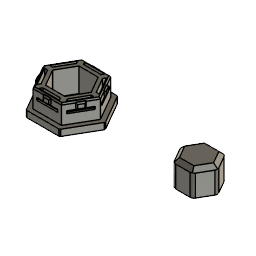
Inserts (Autodesk Fusion 360 design; units mm, degrees)
part number: 2025-05-12-14-06-05-452
part number: 2025-05-25-10-33-36-261
part number: 2025-05-25-10-36-06-309
Autodesk Fusion 360 part; units mm, degrees
sketch "Sketch1" plane through (0, 0, 0) normal (0, 0, 1) x (1, 0, 0)
  line L0 (-6.5818, 11.4) -> (-13.1636, 0)
  line L1 (-13.1636, 0) -> (-6.5818, -11.4)
  line L2 (-6.5818, -11.4) -> (6.5818, -11.4)
  line L3 (6.5818, -11.4) -> (13.1636, 0)
  line L4 (13.1636, 0) -> (6.5818, 11.4)
  line L5 (6.5818, 11.4) -> (-6.5818, 11.4)
  dimension "d1" = 11.4
  measures "d1" distance of origin L5
extrude "Extrude1" add sketch "Sketch1" along normal blind 2.5 makes body 1
sketch "Sketch2" plane through (0, 0, 2.5) normal (0, 0, 1) x (-1, 0, 0)
  line L0 (-6.5818, -11.4) -> (6.5818, -11.4)
  line L1 (6.5818, -11.4) -> (13.1636, 0)
  line L2 (13.1636, 0) -> (6.5818, 11.4)
  line L3 (6.5818, 11.4) -> (-6.5818, 11.4)
  line L4 (-6.5818, 11.4) -> (-13.1636, 0)
  line L5 (-13.1636, 0) -> (-6.5818, -11.4)
  line L6 (5.6003, -9.7) -> (11.2006, 0)
  line L7 (11.2006, 0) -> (5.6003, 9.7)
  line L8 (5.6003, 9.7) -> (-5.6003, 9.7)
  line L9 (-5.6003, 9.7) -> (-11.2006, 0)
  line L10 (-11.2006, 0) -> (-5.6003, -9.7)
  line L11 (-5.6003, -9.7) -> (5.6003, -9.7)
  dimension "d4" = 9.7
  measures "d4" distance of origin L11
extrude "Extrude2" add sketch "Sketch2" along normal blind 7.4 contours L6 L7 L8 L9 L10 L11 bodies 1
sketch "Sketch3" plane through (0, 0, 9.9) normal (0, 0, 1) x (-1, 0, 0)
  line L0 (-5.6003, -9.7) -> (5.6003, -9.7)
  line L1 (5.6003, -9.7) -> (11.2006, 0)
  line L2 (11.2006, 0) -> (5.6003, 9.7)
  line L3 (5.6003, 9.7) -> (-5.6003, 9.7)
  line L4 (-5.6003, 9.7) -> (-11.2006, 0)
  line L5 (-11.2006, 0) -> (-5.6003, -9.7)
  line L6 (3.7816, -6.55) -> (7.5633, 0)
  line L7 (7.5633, 0) -> (3.7816, 6.55)
  line L8 (3.7816, 6.55) -> (-3.7816, 6.55)
  line L9 (-3.7816, 6.55) -> (-7.5633, 0)
  line L10 (-7.5633, 0) -> (-3.7816, -6.55)
  line L11 (-3.7816, -6.55) -> (3.7816, -6.55)
  dimension "d7" = 6.55
  measures "d7" distance of origin L11
extrude "Extrude3" cut sketch "Sketch3" against normal up to surface (9.9 mm away) contours L6 L7 L8 L9 L10 L11 bodies 1
sketch "Sketch4" plane through (0, 0, 9.9) normal (0, 0, 1) x (-1, 0, 0)
  line L0 (-7.5633, 0) -> (-3.7816, 6.55)
  line L1 (-3.7816, 6.55) -> (3.7816, 6.55)
  line L2 (3.7816, 6.55) -> (7.5633, 0)
  line L3 (7.5633, 0) -> (3.7816, -6.55)
  line L4 (3.7816, -6.55) -> (-3.7816, -6.55)
  line L5 (-3.7816, -6.55) -> (-7.5633, 0)
  line L6 (-5.6003, -9.7) -> (5.6003, -9.7)
  line L7 (5.6003, -9.7) -> (11.2006, 0)
  line L8 (11.2006, 0) -> (5.6003, 9.7)
  line L9 (5.6003, 9.7) -> (-5.6003, 9.7)
  line L10 (-5.6003, 9.7) -> (-11.2006, 0)
  line L11 (-11.2006, 0) -> (-5.6003, -9.7)
  line L12 (11.2006, 0) -> (-11.2006, 0) construction
  line L13 (-5.6003, 9.7) -> (5.6003, -9.7) construction
  line L14 (-5.6292, -9.75) -> (5.6292, 9.75) construction
  line L15 (-3.4253, 7.9485) -> (3.431, 7.95)
  line L16 (3.431, 7.95) -> (4.0005, 8.9501)
  line L17 (4.0005, 8.9501) -> (-3.9995, 8.9484)
  line L18 (-3.9995, 8.9484) -> (-3.4253, 7.9485)
  line L19 (3.4049, -7.95) -> (-3.4457, -7.9788)
  line L20 (-3.4457, -7.9788) -> (-4.0185, -8.9812)
  line L21 (-4.0185, -8.9812) -> (3.9815, -8.9476)
  line L22 (3.9815, -8.9476) -> (3.4049, -7.95)
  line L23 (5.1681, 6.9487) -> (8.5549, 0.9746)
  line L24 (8.5549, 0.9746) -> (9.6988, 0.9846)
  line L25 (9.6988, 0.9846) -> (5.7533, 7.944)
  line L26 (5.7533, 7.944) -> (5.1681, 6.9487)
  line L27 (-9.6706, 0.9703) -> (-8.5268, 0.965)
  line L28 (-8.5268, 0.965) -> (-5.1652, 6.9536)
  line L29 (-5.7547, 7.9464) -> (-9.6706, 0.9703)
  line L30 (-5.1652, 6.9536) -> (-5.7547, 7.9464)
  line L31 (-5.1141, -6.9101) -> (-8.6037, -0.9979)
  line L32 (-8.6037, -0.9979) -> (-9.7575, -1.0105)
  line L33 (-9.7575, -1.0105) -> (-5.6911, -7.8999)
  line L34 (-5.6911, -7.8999) -> (-5.1141, -6.9101)
  line L35 (8.5998, -1.0047) -> (5.1477, -6.9347)
  line L36 (9.7535, -1.0105) -> (8.5998, -1.0047)
  line L37 (5.7287, -7.9243) -> (9.7535, -1.0105)
  line L38 (5.1477, -6.9347) -> (5.7287, -7.9243)
  point P0 (-0.0307, 8.5259)
  dimension "d10" = 8
  dimension "d11" = 1
  dimension "d12" = 6.8563
  dimension "d13" = 0.339
  dimension "d14" = 1.4
  dimension "d15" = 8
  dimension "d16" = 1
  dimension "d18" = 1.4
  dimension "d19" = 8
  dimension "d20" = 1
  dimension "d22" = 1.4
  dimension "d23" = 1.0105
  dimension "d24" = 1.0105
  dimension "d25" = 1.0105
  dimension "d26" = 1.0105
  dimension "d27" = 8
  dimension "d28" = 1
  dimension "d30" = 1.4
  dimension "d31" = 1.0105
  dimension "d32" = 8
  dimension "d33" = 1
  dimension "d35" = 1.4
  dimension "d36" = 1.0105
  dimension "d37" = 8
  dimension "d38" = 1
  dimension "d40" = 1.4
  dimension "d41" = 1.0105
  constraint coincident L7.end L8.start
  constraint coincident L10.end L11.start
  constraint coincident L9.end L10.start
  constraint coincident L6.end L7.start
  constraint coincident L6.start L11.end
  constraint coincident L8.end L9.start
  constraint parallel L15 L17
  constraint parallel L19 L21
  constraint parallel L23 L25
  constraint parallel L28 L29
  constraint parallel L31 L33
  constraint parallel L35 L37
  measures "d10" distance of L16.end L17.end
  measures "d11" distance of L15 L17
  measures "d12" horizontal distance of L15.start L15.end
  measures "d13" angle of L14 L16
  measures "d14" distance of L1 L15.end
  measures "d15" distance of L20.end L21.end
  measures "d16" distance of L19 L21
  measures "d18" distance of L4 L19.start
  measures "d19" distance of L24.end L25.end
  measures "d20" distance of L23 L25
  measures "d22" distance of L2 L23.start
  measures "d23" distance of L14 L16.end
  measures "d24" distance of L14 L25.end
  measures "d25" distance of L13 L17.end
  measures "d26" distance of L14 L20.end
  measures "d27" distance of L29.start L27.start
  measures "d28" distance of L28 L29
  measures "d30" distance of L0 L28.end
  measures "d31" distance of L13 L29.start
  measures "d32" distance of L32.end L33.end
  measures "d33" distance of L31 L33
  measures "d35" distance of L5 L31.end
  measures "d36" distance of L12 L32.end
  measures "d37" distance of L37.start L36.start
  measures "d38" distance of L35 L37
  measures "d40" distance of L3 L35.start
  measures "d41" distance of L12 L36.start
  measures "d96" distance of L7.end
extrude "Extrude4" cut sketch "Sketch4" against normal blind 5 contours L15 L16 L17 L18 | L19 L20 L21 L22 | L23 L24 L25 L26 | L27 L28 L29 L30 | L31 L32 L33 L34 | L35 L36 L37 L38 bodies 1
sketch "Sketch5" plane through (0, -9.7, 0) normal (0, -1, 0) x (1, 0, 0)
  line L0 (-5.6003, 2.5) -> (5.6003, 2.5)
  line L1 (5.6003, 2.5) -> (5.6003, 9.9)
  line L2 (5.6003, 9.9) -> (-5.6003, 9.9)
  line L3 (-5.6003, 9.9) -> (-5.6003, 2.5)
  line L4 (0, 9.9) -> (0, 2.5) construction
  line L5 (-5.6003, 6.7) -> (5.6003, 6.7) construction
  line L6 (4.1, 7.2) -> (-4.1, 7.2)
  line L7 (-4.1, 7.2) -> (-4.1, 6.2)
  line L8 (-4.1, 6.2) -> (4.1, 6.2)
  line L9 (4.1, 6.2) -> (4.1, 7.2)
  line L10 (4.1, 7.2) -> (-4.1, 6.2) construction
  line L11 (-4.1, 7.2) -> (4.1, 6.2) construction
  point P0 (0, 6.7)
  dimension "d44" = 3.2
  dimension "d45" = 8.2
  dimension "d46" = 1
  constraint midpoint L2 L4.start
  constraint midpoint L0 L4.end
  constraint coincident L3 L5.start
  constraint coincident L1 L5.end
  constraint perpendicular L1 L5
  constraint horizontal L6
  constraint perpendicular L6 L7
  constraint parallel L6 L8
  constraint parallel L7 L9
  constraint coincident L10 P0
  constraint coincident L11 P0
  constraint midpoint L5 P0
  measures "d44" distance of L2 L5
  measures "d45" distance of L7.end L8.end
  measures "d46" distance of L6.end L7.end
extrude "Extrude5" cut sketch "Sketch5" against normal up to surface (1.7515 mm away) contours L6 L7 L8 L9 bodies 1
sketch "Sketch6" plane through (8.4004, -4.85, 0) normal (0.866025, -0.5, 0) x (0.5, 0.866025, 0)
  line L0 (-5.6003, 2.5) -> (5.6003, 2.5)
  line L1 (5.6003, 2.5) -> (5.6003, 9.9)
  line L2 (5.6003, 9.9) -> (-5.6003, 9.9)
  line L3 (-5.6003, 9.9) -> (-5.6003, 2.5)
  line L4 (0, 9.9) -> (0, 2.5) construction
  line L5 (-5.6003, 6.7) -> (5.6003, 6.7) construction
  line L6 (4.1, 6.2) -> (-4.1, 6.2)
  line L7 (-4.1, 6.2) -> (-4.1, 7.2)
  line L8 (-4.1, 7.2) -> (4.1, 7.2)
  line L9 (4.1, 7.2) -> (4.1, 6.2)
  line L10 (4.1, 6.2) -> (-4.1, 7.2) construction
  line L11 (-4.1, 6.2) -> (4.1, 7.2) construction
  point P0 (0, 6.7)
  dimension "d49" = 3.2
  dimension "d50" = 8.2
  dimension "d51" = 1
  constraint midpoint L2 L4.start
  constraint midpoint L0 L4.end
  constraint coincident L3 L5.start
  constraint coincident L1 L5.end
  constraint perpendicular L1 L5
  constraint horizontal L6
  constraint perpendicular L6 L7
  constraint parallel L6 L8
  constraint parallel L7 L9
  constraint coincident L10 P0
  constraint coincident L11 P0
  constraint midpoint L5 P0
  measures "d49" distance of L2 L5
  measures "d50" distance of L7.end L8.end
  measures "d51" distance of L6.end L7.end
extrude "Extrude6" cut sketch "Sketch6" along normal up to surface contours L6 L7 L8 L9 end surface through (8.5268, -0.965, 9.9) normal (0.872011, -0.489485, 0) offset 0 bodies 1
sketch "Sketch7" plane through (8.4004, 4.85, 0) normal (0.866025, 0.5, 0) x (-0.5, 0.866025, 0)
  line L0 (-5.6003, 2.5) -> (5.6003, 2.5)
  line L1 (5.6003, 2.5) -> (5.6003, 9.9)
  line L2 (5.6003, 9.9) -> (-5.6003, 9.9)
  line L3 (-5.6003, 9.9) -> (-5.6003, 2.5)
  line L4 (0, 9.9) -> (0, 2.5) construction
  line L5 (-5.6003, 6.7) -> (5.6003, 6.7) construction
  line L6 (4.1, 7.2) -> (-4.1, 7.2)
  line L7 (-4.1, 7.2) -> (-4.1, 6.2)
  line L8 (-4.1, 6.2) -> (4.1, 6.2)
  line L9 (4.1, 6.2) -> (4.1, 7.2)
  line L10 (4.1, 7.2) -> (-4.1, 6.2) construction
  line L11 (-4.1, 7.2) -> (4.1, 6.2) construction
  point P0 (0, 6.7)
  dimension "d54" = 3.2
  dimension "d55" = 8.2
  dimension "d56" = 1
  constraint midpoint L2 L4.start
  constraint midpoint L0 L4.end
  constraint coincident L3 L5.start
  constraint coincident L1 L5.end
  constraint perpendicular L1 L5
  constraint horizontal L6
  constraint perpendicular L6 L7
  constraint parallel L6 L8
  constraint parallel L7 L9
  constraint coincident L10 P0
  constraint coincident L11 P0
  constraint midpoint L5 P0
  measures "d54" distance of L2 L5
  measures "d55" distance of L7.end L8.end
  measures "d56" distance of L6.end L7.end
extrude "Extrude7" cut sketch "Sketch7" along normal up to surface contours L6 L7 L8 L9 end surface through (5.1141, 6.9101, 9.9) normal (0.861181, 0.508299, 0) offset 0 bodies 1
sketch "Sketch8" plane through (0, 9.7, 0) normal (0, 1, 0) x (-1, 0, 0)
  line L0 (-5.6003, 2.5) -> (5.6003, 2.5)
  line L1 (5.6003, 2.5) -> (5.6003, 9.9)
  line L2 (5.6003, 9.9) -> (-5.6003, 9.9)
  line L3 (-5.6003, 9.9) -> (-5.6003, 2.5)
  line L4 (0, 9.9) -> (0, 2.5) construction
  line L5 (5.6003, 6.7) -> (-5.6003, 6.7) construction
  line L6 (4.1, 7.2) -> (-4.1, 7.2)
  line L7 (-4.1, 7.2) -> (-4.1, 6.2)
  line L8 (-4.1, 6.2) -> (4.1, 6.2)
  line L9 (4.1, 6.2) -> (4.1, 7.2)
  line L10 (4.1, 7.2) -> (-4.1, 6.2) construction
  line L11 (-4.1, 7.2) -> (4.1, 6.2) construction
  point P0 (0, 6.7)
  dimension "d59" = 3.2
  dimension "d60" = 8.2
  dimension "d61" = 1
  constraint midpoint L2 L4.start
  constraint midpoint L0 L4.end
  constraint coincident L1 L5.start
  constraint coincident L3 L5.end
  constraint perpendicular L3 L5
  constraint horizontal L6
  constraint perpendicular L6 L7
  constraint parallel L6 L8
  constraint parallel L7 L9
  constraint coincident L10 P0
  constraint coincident L11 P0
  constraint midpoint L5 P0
  measures "d59" distance of L2 L5
  measures "d60" distance of L7.end L8.end
  measures "d61" distance of L6.end L7.end
extrude "Extrude8" cut sketch "Sketch8" along normal up to surface contours L6 L7 L8 L9 end surface through (-3.4049, 7.95, 9.9) normal (-0.004199, 0.999991, 0) offset 0 bodies 1
sketch "Sketch9" plane through (-8.4004, 4.85, 0) normal (-0.866025, 0.5, 0) x (-0.5, -0.866025, 0)
  line L0 (-5.6003, 2.5) -> (5.6003, 2.5)
  line L1 (5.6003, 2.5) -> (5.6003, 9.9)
  line L2 (5.6003, 9.9) -> (-5.6003, 9.9)
  line L3 (-5.6003, 9.9) -> (-5.6003, 2.5)
  line L4 (0, 9.9) -> (0, 2.5) construction
  line L5 (5.6003, 6.7) -> (-5.6003, 6.7) construction
  line L6 (4.1, 7.2) -> (-4.1, 7.2)
  line L7 (-4.1, 7.2) -> (-4.1, 6.2)
  line L8 (-4.1, 6.2) -> (4.1, 6.2)
  line L9 (4.1, 6.2) -> (4.1, 7.2)
  line L10 (4.1, 7.2) -> (-4.1, 6.2) construction
  line L11 (-4.1, 7.2) -> (4.1, 6.2) construction
  point P0 (0, 6.7)
  dimension "d64" = 3.2
  dimension "d65" = 8.2
  dimension "d66" = 1
  constraint midpoint L2 L4.start
  constraint midpoint L0 L4.end
  constraint coincident L1 L5.start
  constraint coincident L3 L5.end
  constraint perpendicular L3 L5
  constraint horizontal L6
  constraint perpendicular L6 L7
  constraint parallel L6 L8
  constraint parallel L7 L9
  constraint coincident L10 P0
  constraint coincident L11 P0
  constraint midpoint L5 P0
  measures "d64" distance of L2 L5
  measures "d65" distance of L7.end L8.end
  measures "d66" distance of L6.end L7.end
extrude "Extrude9" cut sketch "Sketch9" along normal up to surface contours L6 L7 L8 L9 end surface through (-8.5998, 1.0047, 9.9) normal (-0.864228, 0.5031, 0) offset 0 bodies 1
sketch "Sketch10" plane through (-8.4004, -4.85, 0) normal (-0.866025, -0.5, 0) x (0.5, -0.866025, 0)
  line L0 (-5.6003, 2.5) -> (5.6003, 2.5)
  line L1 (5.6003, 2.5) -> (5.6003, 9.9)
  line L2 (5.6003, 9.9) -> (-5.6003, 9.9)
  line L3 (-5.6003, 9.9) -> (-5.6003, 2.5)
  line L4 (0, 9.9) -> (0, 2.5) construction
  line L5 (5.6003, 6.7) -> (-5.6003, 6.7) construction
  line L6 (4.1, 7.2) -> (-4.1, 7.2)
  line L7 (-4.1, 7.2) -> (-4.1, 6.2)
  line L8 (-4.1, 6.2) -> (4.1, 6.2)
  line L9 (4.1, 6.2) -> (4.1, 7.2)
  line L10 (4.1, 7.2) -> (-4.1, 6.2) construction
  line L11 (-4.1, 7.2) -> (4.1, 6.2) construction
  point P0 (0, 6.7)
  dimension "d69" = 3.2
  dimension "d70" = 8.2
  dimension "d71" = 1
  constraint midpoint L2 L4.start
  constraint midpoint L0 L4.end
  constraint coincident L1 L5.start
  constraint coincident L3 L5.end
  constraint perpendicular L3 L5
  constraint horizontal L6
  constraint perpendicular L6 L7
  constraint parallel L6 L8
  constraint parallel L7 L9
  constraint coincident L10 P0
  constraint coincident L11 P0
  constraint midpoint L5 P0
  measures "d69" distance of L2 L5
  measures "d70" distance of L7.end L8.end
  measures "d71" distance of L6.end L7.end
extrude "Extrude10" cut sketch "Sketch10" along normal up to surface contours L6 L7 L8 L9 end surface through (-5.1681, -6.9487, 9.9) normal (-0.869926, -0.493182, 0) offset 0 bodies 1
sketch "Sketch11" plane through (0, -9.7, 0) normal (0, -1, 0) x (1, 0, 0)
  line L0 (4.1, 7.2) -> (4.1, 6.2)
  line L1 (4.1, 6.2) -> (-4.1, 6.2)
  line L2 (-4.1, 6.2) -> (-4.1, 7.2)
  line L3 (-4.1, 7.2) -> (4.1, 7.2)
  line L4 (-5.6003, 2.5) -> (5.6003, 2.5)
  line L5 (5.6003, 2.5) -> (5.6003, 9.9)
  line L6 (5.6003, 9.9) -> (-5.6003, 9.9)
  line L7 (-5.6003, 9.9) -> (-5.6003, 2.5)
  line L8 (-5.6003, 8.55) -> (5.6003, 8.55) construction
  line L9 (0, 7.2) -> (0, 9.9) construction
  line L10 (1.55, 9.55) -> (-1.55, 9.55)
  line L11 (-1.55, 9.55) -> (-1.55, 7.55)
  line L12 (-1.55, 7.55) -> (1.55, 7.55)
  line L13 (1.55, 7.55) -> (1.55, 9.55)
  line L14 (1.55, 9.55) -> (-1.55, 7.55) construction
  line L15 (-1.55, 9.55) -> (1.55, 7.55) construction
  point P0 (0, 8.55)
  dimension "d75" = 1.35
  dimension "d76" = 3.1
  dimension "d77" = 2
  constraint coincident L7 L8.start
  constraint coincident L5 L8.end
  constraint perpendicular L5 L8
  constraint midpoint L3 L9.start
  constraint midpoint L6 L9.end
  constraint horizontal L10
  constraint perpendicular L10 L11
  constraint parallel L10 L12
  constraint parallel L11 L13
  constraint coincident L14 P0
  constraint coincident L15 P0
  constraint midpoint L8 P0
  measures "d75" distance of L6 L8
  measures "d76" distance of L11.end L12.end
  measures "d77" distance of L10.end L11.end
extrude "Extrude11" add sketch "Sketch11" along normal blind 0.45 contours L10 L11 L12 L13 bodies 1
sketch "Sketch12" plane through (8.4004, -4.85, 0) normal (0.866025, -0.5, 0) x (0.5, 0.866025, 0)
  line L0 (-4.1, 7.2) -> (4.1, 7.2)
  line L1 (4.1, 7.2) -> (4.1, 6.2)
  line L2 (4.1, 6.2) -> (-4.1, 6.2)
  line L3 (-4.1, 6.2) -> (-4.1, 7.2)
  line L4 (-5.6003, 2.5) -> (5.6003, 2.5)
  line L5 (5.6003, 2.5) -> (5.6003, 9.9)
  line L6 (5.6003, 9.9) -> (-5.6003, 9.9)
  line L7 (-5.6003, 9.9) -> (-5.6003, 2.5)
  line L8 (0, 7.2) -> (0, 9.9) construction
  line L9 (5.6003, 8.55) -> (-5.6003, 8.55) construction
  line L10 (1.55, 7.55) -> (-1.55, 7.55)
  line L11 (-1.55, 7.55) -> (-1.55, 9.55)
  line L12 (-1.55, 9.55) -> (1.55, 9.55)
  line L13 (1.55, 9.55) -> (1.55, 7.55)
  line L14 (1.55, 7.55) -> (-1.55, 9.55) construction
  line L15 (-1.55, 7.55) -> (1.55, 9.55) construction
  point P0 (0, 8.55)
  dimension "d80" = 1.35
  dimension "d81" = 3.1
  dimension "d82" = 2
  constraint midpoint L0 L8.start
  constraint midpoint L6 L8.end
  constraint coincident L5 L9.start
  constraint coincident L7 L9.end
  constraint perpendicular L7 L9
  constraint horizontal L10
  constraint perpendicular L10 L11
  constraint parallel L10 L12
  constraint parallel L11 L13
  constraint coincident L14 P0
  constraint coincident L15 P0
  constraint midpoint L8 P0
  measures "d80" distance of L6 L9
  measures "d81" distance of L11.end L12.end
  measures "d82" distance of L10.end L11.end
extrude "Extrude12" add sketch "Sketch12" along normal blind 0.45 contours L10 L11 L12 L13 bodies 1
sketch "Sketch13" plane through (8.4004, 4.85, 0) normal (0.866025, 0.5, 0) x (-0.5, 0.866025, 0)
  line L0 (4.1, 7.2) -> (4.1, 6.2)
  line L1 (4.1, 6.2) -> (-4.1, 6.2)
  line L2 (-4.1, 6.2) -> (-4.1, 7.2)
  line L3 (-4.1, 7.2) -> (4.1, 7.2)
  line L4 (-5.6003, 2.5) -> (5.6003, 2.5)
  line L5 (5.6003, 2.5) -> (5.6003, 9.9)
  line L6 (5.6003, 9.9) -> (-5.6003, 9.9)
  line L7 (-5.6003, 9.9) -> (-5.6003, 2.5)
  line L8 (0, 9.9) -> (0, 7.2) construction
  line L9 (5.6003, 8.55) -> (-5.6003, 8.55) construction
  line L10 (1.55, 7.55) -> (-1.55, 7.55)
  line L11 (-1.55, 7.55) -> (-1.55, 9.55)
  line L12 (-1.55, 9.55) -> (1.55, 9.55)
  line L13 (1.55, 9.55) -> (1.55, 7.55)
  line L14 (1.55, 7.55) -> (-1.55, 9.55) construction
  line L15 (-1.55, 7.55) -> (1.55, 9.55) construction
  point P0 (0, 8.55)
  dimension "d85" = 1.35
  dimension "d86" = 3.1
  dimension "d87" = 2
  constraint midpoint L6 L8.start
  constraint midpoint L3 L8.end
  constraint coincident L5 L9.start
  constraint coincident L7 L9.end
  constraint perpendicular L7 L9
  constraint horizontal L10
  constraint perpendicular L10 L11
  constraint parallel L10 L12
  constraint parallel L11 L13
  constraint coincident L14 P0
  constraint coincident L15 P0
  constraint midpoint L8 P0
  measures "d85" distance of L6 L9
  measures "d86" distance of L11.end L12.end
  measures "d87" distance of L10.end L11.end
extrude "Extrude13" add sketch "Sketch13" along normal blind 0.45 contours L10 L11 L12 L13 bodies 1
sketch "Sketch14" plane through (0, 9.7, 0) normal (0, 1, 0) x (-1, 0, 0)
  line L0 (4.1, 7.2) -> (4.1, 6.2)
  line L1 (4.1, 6.2) -> (-4.1, 6.2)
  line L2 (-4.1, 6.2) -> (-4.1, 7.2)
  line L3 (-4.1, 7.2) -> (4.1, 7.2)
  line L4 (-5.6003, 2.5) -> (5.6003, 2.5)
  line L5 (5.6003, 2.5) -> (5.6003, 9.9)
  line L6 (5.6003, 9.9) -> (-5.6003, 9.9)
  line L7 (-5.6003, 9.9) -> (-5.6003, 2.5)
  line L8 (0, 7.2) -> (0, 9.9) construction
  line L9 (5.6003, 8.55) -> (-5.6003, 8.55) construction
  line L10 (1.55, 9.55) -> (-1.55, 9.55)
  line L11 (-1.55, 9.55) -> (-1.55, 7.55)
  line L12 (-1.55, 7.55) -> (1.55, 7.55)
  line L13 (1.55, 7.55) -> (1.55, 9.55)
  line L14 (1.55, 9.55) -> (-1.55, 7.55) construction
  line L15 (-1.55, 9.55) -> (1.55, 7.55) construction
  point P0 (0, 8.55)
  dimension "d90" = 1.35
  dimension "d91" = 3.1
  dimension "d92" = 2
  constraint midpoint L3 L8.start
  constraint midpoint L6 L8.end
  constraint coincident L5 L9.start
  constraint coincident L7 L9.end
  constraint perpendicular L7 L9
  constraint horizontal L10
  constraint perpendicular L10 L11
  constraint parallel L10 L12
  constraint parallel L11 L13
  constraint coincident L14 P0
  constraint coincident L15 P0
  constraint midpoint L8 P0
  measures "d90" distance of L6 L9
  measures "d91" distance of L11.end L12.end
  measures "d92" distance of L10.end L11.end
extrude "Extrude14" add sketch "Sketch14" along normal blind 0.45 contours L10 L11 L12 L13 bodies 1
sketch "Sketch15" plane through (-8.4004, 4.85, 0) normal (-0.866025, 0.5, 0) x (-0.5, -0.866025, 0)
  line L0 (4.1, 7.2) -> (4.1, 6.2)
  line L1 (4.1, 6.2) -> (-4.1, 6.2)
  line L2 (-4.1, 6.2) -> (-4.1, 7.2)
  line L3 (-4.1, 7.2) -> (4.1, 7.2)
  line L4 (-5.6003, 2.5) -> (5.6003, 2.5)
  line L5 (5.6003, 2.5) -> (5.6003, 9.9)
  line L6 (5.6003, 9.9) -> (-5.6003, 9.9)
  line L7 (-5.6003, 9.9) -> (-5.6003, 2.5)
  line L8 (0, 9.9) -> (0, 7.2) construction
  line L9 (5.6003, 8.55) -> (-5.6003, 8.55) construction
  line L10 (1.55, 9.55) -> (-1.55, 9.55)
  line L11 (-1.55, 9.55) -> (-1.55, 7.55)
  line L12 (-1.55, 7.55) -> (1.55, 7.55)
  line L13 (1.55, 7.55) -> (1.55, 9.55)
  line L14 (1.55, 9.55) -> (-1.55, 7.55) construction
  line L15 (-1.55, 9.55) -> (1.55, 7.55) construction
  point P0 (0, 8.55)
  dimension "d95" = 1.35
  dimension "d96" = 2
  dimension "d114" = 1.55
  constraint midpoint L6 L8.start
  constraint midpoint L3 L8.end
  constraint coincident L5 L9.start
  constraint coincident L7 L9.end
  constraint perpendicular L7 L9
  constraint horizontal L10
  constraint perpendicular L10 L11
  constraint parallel L10 L12
  constraint parallel L11 L13
  constraint coincident L14 P0
  constraint coincident L15 P0
  constraint midpoint L9 P0
  measures "d95" distance of L6 L9
  measures "d96" distance of L10.end L11.end
  measures "d114" distance of L8 L11
extrude "Extrude15" add sketch "Sketch15" along normal blind 0.45 contours L10 L11 L12 L13 bodies 1
sketch "Sketch16" plane through (-8.4004, -4.85, 0) normal (-0.866025, -0.5, 0) x (0.5, -0.866025, 0)
  line L0 (4.1, 7.2) -> (4.1, 6.2)
  line L1 (4.1, 6.2) -> (-4.1, 6.2)
  line L2 (-4.1, 6.2) -> (-4.1, 7.2)
  line L3 (-4.1, 7.2) -> (4.1, 7.2)
  line L4 (-5.6003, 2.5) -> (5.6003, 2.5)
  line L5 (5.6003, 2.5) -> (5.6003, 9.9)
  line L6 (5.6003, 9.9) -> (-5.6003, 9.9)
  line L7 (-5.6003, 9.9) -> (-5.6003, 2.5)
  line L8 (0, 9.9) -> (0, 7.2) construction
  line L9 (5.6003, 8.55) -> (-5.6003, 8.55) construction
  line L10 (1.55, 7.55) -> (-1.55, 7.55)
  line L11 (-1.55, 7.55) -> (-1.55, 9.55)
  line L12 (-1.55, 9.55) -> (1.55, 9.55)
  line L13 (1.55, 9.55) -> (1.55, 7.55)
  line L14 (1.55, 7.55) -> (-1.55, 9.55) construction
  line L15 (-1.55, 7.55) -> (1.55, 9.55) construction
  point P0 (0, 8.55)
  dimension "d99" = 1.35
  dimension "d100" = 3.1
  dimension "d101" = 2
  constraint midpoint L6 L8.start
  constraint midpoint L3 L8.end
  constraint coincident L5 L9.start
  constraint coincident L7 L9.end
  constraint perpendicular L7 L9
  constraint horizontal L10
  constraint perpendicular L10 L11
  constraint parallel L10 L12
  constraint parallel L11 L13
  constraint coincident L14 P0
  constraint coincident L15 P0
  constraint midpoint L9 P0
  measures "d99" distance of L6 L9
  measures "d100" distance of L11.end L12.end
  measures "d101" distance of L10.end L11.end
extrude "Extrude16" add sketch "Sketch16" along normal blind 0.45 contours L10 L11 L12 L13 bodies 1
fillet "Fillet2" radius 0.5 6 edges at (-13.1636, 0, 1.25) (-6.5818, -11.4, 1.25) (6.5818, -11.4, 1.25) (13.1636, 0, 1.25) (6.5818, 11.4, 1.25) (-6.5818, 11.4, 1.25) on bodies 1
sketch "Sketch17" plane through (0, 0, 0) normal (0, 0, -1) x (1, 0, 0)
  line L0 (3.7816, 6.55) -> (7.5633, 0)
  line L1 (7.5633, 0) -> (3.7816, -6.55)
  line L2 (3.7816, -6.55) -> (-3.7816, -6.55)
  line L3 (-3.7816, -6.55) -> (-7.5633, 0)
  line L4 (-7.5633, 0) -> (-3.7816, 6.55)
  line L5 (-3.7816, 6.55) -> (3.7816, 6.55)
  arc A0 (-6.7261, -11.15) -> (-6.2931, -11.4) centre (-6.2931, -10.9) ccw
  line L6 (-6.2931, -11.4) -> (6.2931, -11.4)
  arc A1 (6.2931, -11.4) -> (6.7261, -11.15) centre (6.2931, -10.9) ccw
  line L7 (6.7261, -11.15) -> (13.0192, -0.25)
  arc A2 (13.0192, -0.25) -> (13.0192, 0.25) centre (12.5862, 0) ccw
  line L8 (13.0192, 0.25) -> (6.7261, 11.15)
  arc A3 (6.7261, 11.15) -> (6.2931, 11.4) centre (6.2931, 10.9) ccw
  line L9 (6.2931, 11.4) -> (-6.2931, 11.4)
  arc A4 (-6.2931, 11.4) -> (-6.7261, 11.15) centre (-6.2931, 10.9) ccw
  line L10 (-6.7261, 11.15) -> (-13.0192, 0.25)
  arc A5 (-13.0192, 0.25) -> (-13.0192, -0.25) centre (-12.5862, 0) ccw
  line L11 (-13.0192, -0.25) -> (-6.7261, -11.15)
  line L12 (-11, 0) -> (-5.5, -9.5263)
  line L13 (-5.5, -9.5263) -> (5.5, -9.5263)
  line L14 (5.5, -9.5263) -> (11, 0)
  line L15 (11, 0) -> (5.5, 9.5263)
  line L16 (5.5, 9.5263) -> (-5.5, 9.5263)
  line L17 (-5.5, 9.5263) -> (-11, 0)
  line L18 (-9.4576, 0) -> (-4.7288, -8.1905)
  line L19 (-4.7288, -8.1905) -> (4.7288, -8.1905)
  line L20 (4.7288, -8.1905) -> (9.4576, 0)
  line L21 (9.4576, 0) -> (4.7288, 8.1905)
  line L22 (4.7288, 8.1905) -> (-4.7288, 8.1905)
  line L23 (-4.7288, 8.1905) -> (-9.4576, 0)
extrude "Extrude17" cut sketch "Sketch17" against normal blind 0.5 contours L12 L13 L14 L15 L16 L17 bodies 1
chamfer "Chamfer1" distance 0.5 angle 45 6 edges at (0, 6.55, 0) (-5.6725, 3.275, 0) (-5.6725, -3.275, 0) (0, -6.55, 0) (5.6725, -3.275, 0) (5.6725, 3.275, 0) on bodies 1
chamfer "Chamfer2" distance 0.5 angle 45 6 edges at (0, -9.7, 9.9) (8.4004, -4.85, 9.9) (-8.4004, -4.85, 9.9) (-8.4004, 4.85, 9.9) (0, 9.7, 9.9) (8.4004, 4.85, 9.9) on bodies 1
chamfer "Chamfer3" distance 0.5 angle 45 18 edges at (0, -10.15, 9.55) (-1.55, -10.15, 8.55) (1.55, -10.15, 8.55) (8.7902, -5.075, 9.55) (8.0152, -6.4173, 8.55) (9.5652, -3.7327, 8.55) (9.5652, 3.7327, 8.55) (8.7902, 5.075, 9.55) (8.0152, 6.4173, 8.55) (1.55, 10.15, 8.55) (0, 10.15, 9.55) (-1.55, 10.15, 8.55) (-8.0152, 6.4173, 8.55) (-8.7902, 5.075, 9.55) (-9.5652, 3.7327, 8.55) (-9.5652, -3.7327, 8.55) (-8.7902, -5.075, 9.55) (-8.0152, -6.4173, 8.55) on bodies 1
copy_body "Body->Comp1" bodies 1 removing the originals makes body 2 in component "Anchor Insert"
sketch "Sketch1 (2)" plane through (0, 0, 0) normal (0, 0, 1) x (1, 0, 0) in component "Core Insert"
  line L0 (57.4, 0) -> (53.7, 6.4086)
  line L1 (53.7, 6.4086) -> (46.3, 6.4086)
  line L2 (46.3, 6.4086) -> (42.6, 0)
  line L3 (42.6, 0) -> (46.3, -6.4086)
  line L4 (46.3, -6.4086) -> (53.7, -6.4086)
  line L5 (53.7, -6.4086) -> (57.4, 0)
  point P0 (50, 0)
  dimension "d116" = 7.4
  measures "d116" distance of L0.start P0
extrude "Extrude1'" add sketch "Sketch1 (2)" along normal blind 10 separate body makes body 3 in component "Core Insert"
chamfer "Chamfer1'" distance 1.5 angle 45 6 edges at (50, 6.4086, 10) (44.45, 3.2043, 10) (44.45, -3.2043, 10) (50, -6.4086, 10) (55.55, -3.2043, 10) (55.55, 3.2043, 10) on bodies 3 in component "Core Insert"
fillet "Fillet1" radius 1.5 6 edges at (42.6, 0, 4.25) (46.3, -6.4086, 4.25) (53.7, -6.4086, 4.25) (57.4, 0, 4.25) (53.7, 6.4086, 4.25) (46.3, 6.4086, 4.25) on bodies 3 in component "Core Insert"
component "Anchor Insert" placed x (1, 0, 0) y (0, 1, 0) z (0, 0, 1) at (0, 0, 0)
component "Core Insert" placed x (1, 0, 0) y (0, 1, 0) z (0, 0, 1) at (0, 0, 0)
equation "d1 = ( 22.8 / 2 ) * 1 mm"
equation "d5 = 10.1 mm - 2.7 mm"
equation "d7 = ( 13.1 / 2 ) * 1 mm"
equation "d44 = 2.7 mm + 0.5 mm"
equation "d75 = ( 2.7 / 2 ) * 1 mm"
equation "d114 = ( 3.1 / 2 ) * 1 mm"
